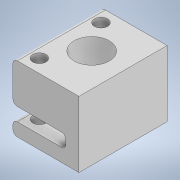
# Autodesk Inventor part: support tige voiture
Saved by Autodesk Inventor 2020.2 (Build 242310000, 310)
## iProperties
Created: 2020-02-28
Part Number: support tige voiture
Material: Générique
Document SubType Name: Modeling
Designer: anton
Density: 1 g/cm^3
Appearance: Par défaut
Author: anton
Autodesk Inventor part; units mm, degrees
ref_plane "YZ Plane" through (0, 0, 0) normal (1, 0, 0) x (0, 1, 0)
ref_plane "XZ Plane" through (0, 0, 0) normal (0, 1, 0) x (-1, 0, 0)
ref_plane "XY Plane" through (0, 0, 0) normal (0, 0, 1) x (1, 0, 0)
sketch "Esquisse1" plane through (0, 0, 0) normal (0, 0, 1) x (1, 0, 0)
  line L0 (-24.5097, 12.7546) -> (-9.5097, 12.7546)
  line L1 (-9.5097, 12.7546) -> (-9.5097, -2.2454)
  line L2 (-9.5097, -2.2454) -> (-24.5097, -2.2454)
  line L3 (-24.5097, -2.2454) -> (-24.5097, 0.7546)
  line L4 (-24.5097, 0.7546) -> (-12.5097, 0.7546)
  line L5 (-12.5097, 0.7546) -> (-12.5097, 3.7546)
  line L6 (-12.5097, 3.7546) -> (-24.5097, 3.7546)
  line L7 (-24.5097, 3.7546) -> (-24.5097, 12.7546)
  dimension "d0" = 15
  dimension "d1" = 15
  dimension "d2" = 3
  dimension "d3" = 9
  dimension "d4" = 12
  constraints: 16 end point, 7 perpendicular, 1 horizontal, 1 point on line
  measures "d0" distance of L0.start L0.end
  measures "d1" distance of L0.end L1.end
  measures "d2" distance of L4.end L5.end
  measures "d3" distance of L6.end L0.start
  measures "d4" distance of L5.end L6.end
extrude "Extrusion1" add sketch "Esquisse1" along normal blind 20
sketch "Esquisse2" plane through (-24.5097, 12.7546, 0) normal (0, 1, 0) x (1, 0, 0)
  circle A0 centre (3, -3) radius 1.5
  circle A1 centre (3, -17) radius 1.5
  line L0 (0, 0) -> (0, -20) projected
  line L1 (15, 0) -> (0, 0) projected
  line L2 (15, -20) -> (0, -20) projected
  point P0 (24.5097, 0)
  dimension "d8" = 3
  dimension "d9" = 3
  dimension "d13" = 3
  dimension "d15" = 3
  dimension "d30" = 3
  dimension "d31" = 3
  constraints: 2 centre point
  measures "d8" distance from line of L0 A0.centre
  measures "d9" diameter of A0
  measures "d13" distance from line of L0 A1.centre
  measures "d15" diameter of A1
  measures "d30" distance from line of L1 A0.centre
  measures "d31" distance from line of L2 A1.centre
hole "Perçage1" at (-21.5097, 12.7546, 3) at (-21.5097, 12.7546, 17) direction (0, -1, 0) diameter 3 end through all
sketch "Esquisse3" plane through (-24.5097, 12.7546, 0) normal (0, 1, 0) x (1, 0, 0)
  circle A0 centre (7.5, -9.6122) radius 4
  line L0 (15, 0) -> (15, -20) projected
  point P0 (24.5097, 0)
  dimension "d26" = 8
  dimension "d27" = 7.5
  constraints: 1 centre point
  measures "d26" diameter of A0
  measures "d27" distance from line of A0.centre L0
extrude "Extrusion2" cut sketch "Esquisse3" against normal blind 7
fillet "Congé1" radius 1 6 edges at (-12.5097, 3.7546, 10) (-12.5097, 0.7546, 10) (-24.5097, -2.2454, 10) (-24.5097, 0.7546, 10) (-24.5097, 3.7546, 10) (-24.5097, 12.7546, 10)
